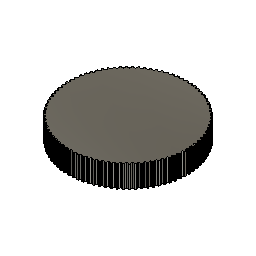
gear_86z (Autodesk Fusion 360 design; units mm, degrees)
Autodesk Fusion 360 part; units mm, degrees
sketch "Sketch1" plane through (0, 0, 0) normal (0, 0, 1) x (1, 0, 0) in component "gt2 pulley"
  circle A0 centre (0, 0) radius 27.3747 construction
  circle A1 centre (0, 0) radius 26.3707 construction
  line L0 (0, 0) -> (0, 27.3747) construction
  line L1 (0, 0) -> (0.9998, 27.3564) construction
  line L2 (0, 0) -> (1.4046, 27.3386) construction
  circle A2 centre (0, 0) radius 27.1207 construction
  arc A3 (0.3966, 26.9846) -> (0.4743, 26.6866) centre (1.3916, 27.0849) ccw
  circle A4 centre (0, 0) radius 26.9707 construction
  arc A5 (0.2487, 27.1195) -> (0, 27.1207) centre (0, 0) ccw
  arc A6 (0.3966, 26.9846) -> (0.2487, 27.1195) centre (0.2474, 26.9695) ccw
  arc A7 (0.4743, 26.6866) -> (0.9631, 26.3531) centre (0.9834, 26.9077) ccw
  arc A8 (0, 27.1207) -> (-0.2487, 27.1195) centre (0, 0) ccw
  arc A9 (-0.2487, 27.1195) -> (-0.3966, 26.9846) centre (-0.2474, 26.9695) ccw
  arc A10 (-0.4743, 26.6866) -> (-0.3966, 26.9846) centre (-1.3916, 27.0849) ccw
  arc A11 (-0.9629, 26.3531) -> (-0.4743, 26.6866) centre (-0.9834, 26.9077) ccw
  arc A12 (0.9631, 26.3531) -> (-0.9631, 26.3531) centre (0, 0) ccw
  point P0 (1.3916, 27.0849)
  point P1 (0, 27.1207)
  dimension "d18" = 54.7493
  dimension "d19" = 2.093
  dimension "d22" = 1.004
  dimension "d24" = 0.75
  dimension "d26" = 1
  dimension "d27" = 0.15
  dimension "d28" = 0.15
  dimension "d47" = 0.555
  dimension "d52" = 3.812
  constraint coincident A0.centre A1.centre
  constraint coincident A0 L0.end
  constraint vertical L0
  constraint coincident A0 L1.end
  constraint coincident A0 L2.end
  constraint concentric A1 A2
  constraint coincident A1 A7.end
  constraint coincident L1 A7.end
  constraint coincident A2 P0
  constraint coincident L2 P0
  constraint coincident P0 A3.centre
  constraint coincident A2 P1
  constraint coincident L0 P1
  constraint concentric A2 A4
  constraint coincident P1 A5.end
  constraint coincident A4 A6.centre
  constraint coincident A3.start A6.start
  constraint tangent A3 A6
  constraint tangent A3 A7
  constraint symmetric L0 A7.end A12.end
  constraint symmetric L0 A3.start A9.end
  constraint symmetric L0 A3.end A10.start
  constraint symmetric L0 A3 A10
  constraint symmetric L0 A5.start A8.end
  constraint symmetric L0 P1 A5.end
  constraint symmetric L0 A5 A8
  constraint symmetric L0 A6 A9
  constraint symmetric L0 A7 A11
  constraint coincident A1 A11.start
  constraint tangent A1 A7
  constraint coincident L1 A7.centre
  measures "d18" diameter of A0
  measures "d19" angle of L0 L1
  measures "d22" distance of A0 A1
  measures "d24" distance of A1 A2
  measures "d26" radius of A3
  measures "d27" distance of A2 A4
  measures "d28" radius of A6
  measures "d47" radius of A7
extrude "Extrude1" add sketch "Sketch1" along normal blind 10 makes body 1
pattern_circular "C-Pattern1" count 86 over 360 about axis through (0, 0, 1.75) along (0, 0, 1) of bodies 1 makes body 2 at (-2.4581, 26.2558, 6.6667) makes body 3 at (-3.0969, 26.1882, 3.3333) makes body 4 at (-5.0002, 25.8923, 3.3333) makes body 5 at (-6.8769, 25.4582, 6.6667) makes body 6 at (-9.5202, 24.5922, 6.6667) makes body 7 at (-10.5103, 24.1856, 3.3333) makes body 8 at (-12.9994, 22.944, 6.6667) makes body 9 at (-13.9198, 22.3976, 3.3333) makes body 10 at (-16.7034, 20.4061, 6.6667) makes body 11 at (-17.0326, 20.1321, 3.3333) makes body 12 at (-19.0584, 18.226, 6.6667) makes body 13 at (-20.7407, 16.2861, 6.6667) makes body 14 at (-21.8741, 14.7287, 6.6667) makes body 15 at (-22.8909, 13.0927, 6.6667) makes body 16 at (-23.1005, 12.7192, 3.3333) makes body 17 at (-24.5533, 9.6202, 6.6667) makes body 18 at (-25.19, 7.8022, 6.6667) makes body 19 at (-25.54, 6.5665, 6.6667) makes body 20 at (-26.0576, 4.0514, 6.6667) makes body 21 at (-26.2239, 2.7779, 6.6667) makes body 22 at (-26.3151, 1.7114, 3.3333) makes body 23 at (-26.3489, -1.07, 6.6667) makes body 24 at (-26.2005, -2.9905, 6.6667) makes body 25 at (-26.0576, -4.0512, 6.6667) makes body 26 at (-25.3134, -7.392, 6.6667) makes body 27 at (-24.9235, -8.6157, 6.6667) makes body 28 at (-24.5533, -9.62, 6.6667) makes body 29 at (-23.1006, -12.719, 6.6667) makes body 30 at (-22.891, -13.0925, 3.3333) makes body 31 at (-21.0025, -15.947, 6.6667) makes body 32 at (-20.2011, -16.9507, 6.6667) makes body 33 at (-18.9099, -18.38, 6.6667) makes body 34 at (-17.6773, -19.5685, 6.6667) makes body 35 at (-16.7035, -20.406, 3.3333) makes body 36 at (-14.1013, -22.2837, 6.6667) makes body 37 at (-12.8129, -23.0487, 6.6667) makes body 38 at (-11.867, -23.5496, 3.3333) makes body 39 at (-10.1163, -24.353, 6.6667) makes body 40 at (-6.8771, -25.4581, 6.6667) makes body 41 at (-5.6293, -25.7628, 6.6667) makes body 42 at (-3.7338, -26.105, 6.6667) makes body 43 at (-1.8183, -26.3079, 6.6667) makes body 44 at (0.1069, -26.3704, 6.6667) makes body 45 at (1.177, -26.3444, 6.6667) makes body 46 at (3.0969, -26.1882, 3.3333) makes body 47 at (5.8381, -25.7163, 6.6667) makes body 48 at (6.8769, -25.4582, 6.6667) makes body 49 at (9.5202, -24.5922, 6.6667) makes body 50 at (10.5103, -24.1856, 3.3333) makes body 51 at (13.5542, -22.6207, 6.6667) makes body 52 at (13.9198, -22.3976, 3.3333) makes body 53 at (16.7034, -20.4061, 6.6667) makes body 54 at (17.5177, -19.7114, 6.6667) makes body 55 at (18.4567, -18.8351, 3.3333) makes body 56 at (20.7407, -16.2861, 6.6667) makes body 57 at (21.8741, -14.7287, 6.6667) makes body 58 at (22.8909, -13.0927, 6.6667) makes body 59 at (23.1005, -12.7192, 3.3333) makes body 60 at (24.5533, -9.6202, 6.6667) makes body 61 at (25.19, -7.8022, 6.6667) makes body 62 at (25.6923, -5.9427, 6.6667) makes body 63 at (26.0576, -4.0514, 6.6667) makes body 64 at (26.2838, -2.1385, 6.6667) makes body 65 at (26.3151, -1.7114, 3.3333) makes body 66 at (26.3489, 1.07, 6.6667) makes body 67 at (26.12, 3.6275, 6.6667) makes body 68 at (26.0576, 4.0512, 6.6667) makes body 69 at (25.4859, 6.7734, 6.6667) makes body 70 at (24.7063, 9.22, 6.6667) makes body 71 at (24.5533, 9.62, 6.6667) makes body 72 at (23.4034, 12.1528, 6.6667) makes body 73 at (22.891, 13.0925, 3.3333) makes body 74 at (21.0025, 15.947, 6.6667) makes body 75 at (20.7408, 16.2859, 3.3333) makes body 76 at (18.4568, 18.835, 6.6667) makes body 77 at (17.6773, 19.5685, 6.6667) makes body 78 at (16.7035, 20.406, 3.3333) makes body 79 at (14.1013, 22.2837, 6.6667) makes body 80 at (13.5544, 22.6206, 3.3333) makes body 81 at (10.5105, 24.1855, 6.6667) makes body 82 at (9.5204, 24.5921, 6.6667) makes body 83 at (6.8771, 25.4581, 6.6667) makes body 84 at (5.6293, 25.7628, 6.6667) makes body 85 at (3.097, 26.1882, 6.6667) makes body 86 at (2.6713, 26.235, 3.3333)
sketch "Sketch2" plane through (0, 0, 10) normal (0, 0, 1) x (-1, 0, 0)
  arc A0 (-8.154, -25.7262) -> (-8.0512, -25.898) centre (-8.0068, -25.7548) ccw
  arc A1 (-8.0512, -25.898) -> (-7.575, -26.0413) centre (0, 0) ccw
  arc A2 (-7.575, -26.0413) -> (-7.3944, -25.9547) centre (-7.533, -25.8973) ccw
  arc A3 (-7.2342, -25.6918) -> (-7.3944, -25.9547) centre (-6.4706, -26.3374) ccw
  arc A4 (-6.6702, -25.5131) -> (-7.2342, -25.6918) centre (-6.8104, -26.0501) ccw
  arc A5 (-8.5146, -24.9582) -> (-6.6702, -25.5131) centre (0, 0) ccw
  arc A6 (-8.1426, -25.4185) -> (-8.5146, -24.9582) centre (-8.6938, -25.4835) ccw
  arc A7 (-8.154, -25.7262) -> (-8.1426, -25.4185) centre (-9.1357, -25.5356) ccw
  circle A8 centre (0, 0) radius 26.3707
  constraint concentric A1 A8
extrude "Extrude2" add sketch "Sketch2" against normal blind 10 contours A5 A8 bodies 1 2 3 4 5 6 7 8 9 10 11 12 13 14 15 16 17 18 19 20 21 22 23 24 25 26 27 28 29 30 31 32 33 34 35 36 37 38 39 40 41 42 43 44 45 46 47 48 49 50 51 52 53 54 55 56 57 58 59 60 61 62 63 64 65 66 67 68 69 70 71 72 73 74 75 76 77 78 79 80 81 82 83 84 85 86
extrude "Extrude4" [suppressed] in component "gt2 pulley"
pattern_circular "C-Pattern7" [suppressed] in component "gt2 pulley"
extrude "Extrude3" [suppressed] in component "gt2 pulley"
pattern_circular "C-Pattern6" [suppressed] in component "gt2 pulley"
extrude "Extrude2'" [suppressed] in component "gt2 pulley"
pattern_circular "C-Pattern5" [suppressed] in component "gt2 pulley"
extrude "Extrude1'" [suppressed] in component "gt2 pulley"
pattern_circular "C-Pattern4" [suppressed] in component "gt2 pulley"
pattern_circular "C-Pattern3" [suppressed] in component "gt2 pulley"
pattern_circular "C-Pattern2" [suppressed] in component "gt2 pulley"
pattern_circular "C-Pattern1'" [suppressed] in component "gt2 pulley"
copy_body "Body->Comp1" [suppressed] in component "Component"
copy_body "Body->Comp2" [suppressed] in component "Component'"
copy_body "Body->Comp3" [suppressed] in component "Component''"
copy_body "Body->Comp4" [suppressed] in component "Component'''"
copy_body "Body->Comp5" [suppressed] in component "Component''''"
copy_body "Body->Comp6" [suppressed] in component "Component'''''"
copy_body "Body->Comp7" [suppressed] in component "Component''''''"
copy_body "Body->Comp8" [suppressed] in component "Component'''''''"
copy_body "Body->Comp9" [suppressed] in component "Component''''''''"
copy_body "Body->Comp10" [suppressed] in component "Component'''''''''"
copy_body "Body->Comp11" [suppressed] in component "Component''''''''''"
copy_body "Body->Comp12" [suppressed] in component "Component'''''''''''"
copy_body "Body->Comp13" [suppressed] in component "Component''''''''''''"
copy_body "Body->Comp14" [suppressed] in component "Component'''''''''''''"
copy_body "Body->Comp15" [suppressed] in component "Component''''''''''''''"
copy_body "Body->Comp16" [suppressed] in component "Component'''''''''''''''"
copy_body "Body->Comp17" [suppressed] in component "Component''''''''''''''''"
copy_body "Body->Comp18" [suppressed] in component "Component'''''''''''''''''"
copy_body "Body->Comp19" [suppressed] in component "Component''''''''''''''''''"
copy_body "Body->Comp20" [suppressed] in component "Component'''''''''''''''''''"
component "gt2 pulley" placed x (1, 0, 0) y (0, 1, 0) z (0, 0, 1) at (0, 0, 0)
equation "NumTeeth = 86" comment "min 20"
equation "ToothPitch = 2 mm"
equation "PullyDia = NumTeeth * ToothPitch / PI"
equation "ToothAng = ( ( 360 / NumTeeth ) * 1 deg )"
equation "TransOffsetAngle = ToothAng * 0.2"
equation "Sholulder_Radius = 0.15 mm"
equation "Root_Radius = 0.555 mm"
equation "TransRadius = 1 mm"
equation "ToolHeight = 0.75 mm"
equation "PLD = 0.254 mm"
equation "d18 = PullyDia"
equation "d19 = ToothAng / 2"
equation "d22 = PLD + ToolHeight"
equation "d24 = ToolHeight"
equation "d26 = TransRadius"
equation "d27 = Sholulder_Radius"
equation "d31 = NumTeeth"
equation "d33 = NumTeeth"
equation "d35 = NumTeeth"
equation "d37 = NumTeeth"
equation "d41 = NumTeeth"
equation "d45 = NumTeeth"
equation "d47 = Root_Radius"
equation "d50 = NumTeeth"
